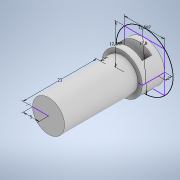
# Autodesk Inventor part: resorte3
Saved by Autodesk Inventor 2021.5 (Build 255421000, 421)
## iProperties
Created: 2024-11-28
Part Number: resorte3
Material: Genérico
Document SubType Name: Modeling
Designer: Joho_
Density: 1 g/cm^3
Appearance: Valor por defecto
Author: Joho_
## iProperties of the stored document _3DPrint.ipt
Created: 2024-11-28
Part Number: _3DPrint
Material: Genérico
Document SubType Name: Modeling
Designer: Joho_
Density: 1 g/cm^3
Appearance: Valor por defecto
Author: Joho_
Autodesk Inventor part; units mm, degrees
ref_plane "YZ Plane" through (0, 0, 0) normal (1, 0, 0) x (0, 1, 0)
ref_plane "XZ Plane" through (0, 0, 0) normal (0, 1, 0) x (-1, 0, 0)
ref_plane "XY Plane" through (0, 0, 0) normal (0, 0, 1) x (1, 0, 0)
sketch "Boceto1" plane through (0, 0, 0) normal (0, 0, 1) x (1, 0, 0)
  circle A0 centre (0, 0) radius 8.9
  line L0 (6.2933, -6.2933) -> (-6.2933, -6.2933)
  line L1 (-6.2933, -6.2933) -> (-6.2933, 6.2933)
  line L2 (-6.2933, 6.2933) -> (6.2933, 6.2933)
  line L3 (6.2933, 6.2933) -> (6.2933, -6.2933)
  dimension "d0" = 17.8
  dimension "d1" = 12.5865
  dimension "d2" = 12.5865
  constraints: 8 end point, 2 parallel, 1 centre point, 1 coincident, 1 horizontal, 1 perpendicular
  measures "d0" diameter of A0
  measures "d1" distance of L1.end L2.end
  measures "d2" distance of L0.end L1.end
sketch "Boceto2" plane through (0, 0, 0) normal (0, 1, 0) x (-1, 0, 0)
  line L0 (6.2933, 0) -> (-6.2933, 0)
  line L1 (-6.2933, 0) -> (-6.2933, 2)
  line L2 (-6.2933, 2) -> (6.2933, 2)
  line L3 (6.2933, 2) -> (6.2933, 0)
  line L4 (-6.2933, 0) -> (6.2933, 0)
  line L5 (6.2933, 0) -> (4.2933, 0)
  line L6 (4.2933, 0) -> (4.2933, 7)
  line L7 (4.2933, 7) -> (6.2933, 7)
  line L8 (6.2933, 7) -> (6.2933, 0)
  line L9 (-6.2933, 0) -> (-4.2933, 0)
  line L10 (-4.2933, 0) -> (-4.2933, 7)
  line L11 (-4.2933, 7) -> (-6.2933, 7)
  line L12 (-6.2933, 7) -> (-6.2933, 0)
  line L13 (-6.2933, 7) -> (6.2933, 7)
  line L14 (6.2933, 7) -> (6.2933, 5)
  line L15 (6.2933, 5) -> (-6.2933, 5)
  line L16 (-6.2933, 5) -> (-6.2933, 7)
  line L17 (0, 7) -> (5, 7)
  line L18 (5, 7) -> (5, 30)
  line L19 (5, 30) -> (0, 30)
  line L20 (0, 30) -> (0, 7)
  line L21 (0, 7) -> (0, 0)
  point P0 (6.2933, 10)
  point P1 (6.2933, 15)
  point P2 (6.2933, 20)
  point P3 (6.2933, 25)
  point P4 (6.2933, 30)
  point P5 (4.2933, 2)
  point P6 (-4.2933, 2)
  point P7 (0, 5)
  point P8 (4.2933, 5)
  point P9 (0, 2)
  point P10 (-4.2933, 5)
  dimension "d5" = 2
  dimension "d28" = 2
  dimension "d29" = 5
  dimension "d30" = 23
  constraints: 44 end point, 4 parallel, 3 perpendicular, 2 horizontal, 1 midpoint
  measures "d5" distance of L0.end L1.end
  measures "d28" distance of L13.end L14.end
  measures "d29" distance of L19.end L18.end
  measures "d30" distance of L18.end L17.end
revolve "Revolución1" add sketch "Boceto2" angle 360 about axis through (0, 0, 7) along (0, 0, -1) contours L0 L6 L2 L3 | L0 L21 L2 L6 | L2 L6 L15 L8 | L15 L6 L7 L8 | L15 L21 L13 L6 | L13 L20 L19 L18 L7
extrude "Extrusión4" cut sketch "Boceto2" against normal mid plane 20 contours L2 L21 L15 L6 | L2 L10 L15 L21
sketch "Boceto4" plane through (0, 0, 0) normal (0, 0, -1) x (-1, 0, 0)
  circle A0 centre (0, 0) radius 2
  dimension "d34" = 4
  constraints: 1 centre point, 1 coincident
  measures "d34" diameter of A0
extrude "Extrusión5" cut sketch "Boceto4" against normal blind 20
chamfer "Chaflán1" distance 2 angle 45 1 edges at (2, 0, 20)
